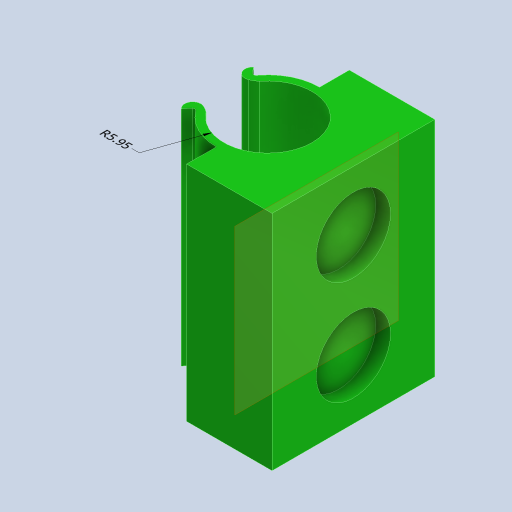
# Autodesk Inventor part: крепление маркера 11мм
Saved by Autodesk Inventor 2024.2 (Build 282272000, 272)
## iProperties
Created: 2025-12-12
Part Number: крепление маркера 11мм
Material: Типовые
Document SubType Name: Modeling
Designer: katya_notebook
Density: 1 g/cm^3
Appearance: Темно-зеленый
Author: katya_notebook
Autodesk Inventor part; units mm, degrees
ref_plane "YZ Plane" through (0, 0, 0) normal (1, 0, 0) x (0, 1, 0)
ref_plane "XZ Plane" through (0, 0, 0) normal (0, 1, 0) x (-1, 0, 0)
ref_plane "XY Plane" through (0, 0, 0) normal (0, 0, 1) x (1, 0, 0)
sketch "Эскиз1" plane through (0, 0, 0) normal (0, 1, 0) x (-1, 0, 0)
  circle A0 centre (0, 0) radius 5.95
  circle A1 centre (0, 0) radius 6.95
  line L0 (0, 0) -> (5.546, 4.1887)
  line L1 (0, 0) -> (5.546, -4.1887)
  point P0 (4.748, -3.586)
  point P1 (4.748, 3.586)
  dimension "d0" = 11.9
  dimension "d1" = 13.9
  constraints: 4 end point, 2 centre point, 2 coincident, 2 point on circle
  measures "d0" diameter of A0
  measures "d1" diameter of A1
extrude "Выдавливание1" add sketch "Эскиз1" along normal blind 30 contours A0 L1 A1 L0 picked at (4.878, 4.401)
sketch "Эскиз2" plane through (0, 30, 0) normal (0, 1, 0) x (1, 0, 0)
  arc A0 (-4.748, -3.586) -> (-5.6407, -3.0561) centre (-7.4493, -7.1199) ccw
  arc A1 (-5.6407, -3.0561) -> (-6.7976, -4.8618) centre (-6.075, -4.0513) ccw
  line L0 (-6.7976, -4.8618) -> (-6.1263, -4.0074)
  arc A2 (-5.5474, -4.1741) -> (-6.1263, -4.0074) centre (-5.9157, -4.3645) ccw
  line L1 (-4.748, -3.586) -> (-5.546, -4.1887)
  line L2 (-5.546, -4.1887) -> (-4.748, -3.586)
  line L3 (-5.546, -4.1887) -> (-5.5474, -4.1741)
  line L4 (-0.0151, 0) -> (-3.489, 0)
  arc A3 (-5.6407, 3.0561) -> (-4.748, 3.586) centre (-7.4493, 7.1199) ccw
  arc A4 (-6.1263, 4.0074) -> (-5.5474, 4.1741) centre (-5.9157, 4.3645) ccw
  line L5 (-4.748, 3.586) -> (-5.546, 4.1887)
  line L6 (-5.546, 4.1887) -> (-4.748, 3.586)
  line L7 (-5.546, 4.1887) -> (-5.5474, 4.1741)
  arc A5 (-6.7976, 4.8618) -> (-5.6407, 3.0561) centre (-6.075, 4.0513) ccw
  line L8 (-6.7976, 4.8618) -> (-6.1263, 4.0074)
  point P0 (-4.748, 3.586)
  point P1 (-5.546, -4.1887)
  point P2 (-5.3694, -4.0591)
  point P3 (-5.3694, 4.0591)
  dimension "d25" = 1.0859
  constraints: 18 end point, 12 point on circle, 12 symmetric about line, 6 centre point, 4 coincident, 1 collinear, 1 horizontal, 3 other
  measures "d25" radius of A1
sketch "Эскиз3" plane through (0, 30, 0) normal (0, 1, 0) x (1, 0, 0)
  arc A0 (-5.546, -4.1887) -> (-5.546, 4.1887) centre (0, 0) ccw projected
  line L0 (11.5, -6.95) -> (11.5, 6.95)
  arc A1 (-4.748, -3.586) -> (-4.748, 3.586) centre (0, 0) ccw projected
  line L1 (0, -6.95) -> (0, -5.95)
  line L2 (0, 5.95) -> (0, 6.95)
  line L3 (11.5, 6.95) -> (11.5, 10.95)
  line L4 (11.5, -6.95) -> (11.5, -10.95)
  line L5 (0, 2.45) -> (0, 6.95)
  line L6 (11.5, -10.95) -> (0, -10.95)
  line L7 (0, -10.95) -> (0, -6.95)
  line L8 (11.5, 10.95) -> (0, 10.95)
  line L9 (0, 10.95) -> (0, 6.95)
  arc A2 (0, -5.95) -> (0, 5.95) centre (0, 0) ccw
  dimension "d13" = 4
  dimension "d14" = 4
  dimension "d22" = 21.9
  dimension "d23" = 5
  constraints: 20 end point, 6 point on circle, 4 vertical, 2 horizontal, 2 perpendicular, 1 centre point, 1 collinear, 1 concentric
  measures "d13" distance of L4.end L0.start
  measures "d14" distance of L3.end L0.end
  measures "d22" distance of L4.end L3.end
  measures "d23" distance of L6.end L1.end
extrude "Выдавливание3" add sketch "Эскиз3" against normal blind 30
ref_plane "РабПлоскость1" through (11.5, 20, 4.95) normal (1, 0, 0) x (0, 0, -1)
sketch "Эскиз4" plane through (11.5, 20, 4.95) normal (1, 0, 0) x (0, 0, -1)
  line L0 (4.95, -20) -> (4.95, 10)
  line L1 (1, 10) -> (8.9, 10) projected
  circle A0 centre (4.95, -12) radius 5
  line L2 (14.4, -20) -> (-4.5, -20) projected
  circle A1 centre (4.95, 2) radius 5
  line L3 (-4.5, 10) -> (14.4, 10) projected
  point P0 (7.3306, 10)
  point P1 (2.5694, 10)
  point P2 (4.95, 10)
  dimension "d15" = 10
  dimension "d16" = 8
  dimension "d17" = 10
  dimension "d18" = 8
  constraints: 3 midpoint, 2 centre point, 2 end point, 2 point on line
  measures "d15" diameter of A0
  measures "d16" distance of A0.centre point (4.95, -20)
  measures "d17" diameter of A1
  measures "d18" distance of point (4.95, 10) A1.centre
extrude "Выдавливание4" cut sketch "Эскиз4" against normal blind 2
extrude "Выдавливание5" add sketch "Эскиз2" against normal blind 30
sketch "Эскиз5" plane through (0, 30, 0) normal (0, 1, 0) x (1, 0, 0)
  arc A0 (0, 6.95) -> (-5.546, 4.1887) centre (0, 0) ccw projected
  line L0 (-5.546, 4.1887) -> (-5.5474, 4.1741) projected
  arc A1 (-6.1263, 4.0074) -> (-5.5474, 4.1741) centre (-5.9157, 4.3645) ccw projected
  line L1 (-6.1263, 4.0074) -> (-6.7976, 4.8618) projected
  arc A2 (-6.7976, 4.8618) -> (-5.6407, 3.0561) centre (-6.075, 4.0513) ccw projected
  arc A3 (-5.6407, 3.0561) -> (-4.748, 3.586) centre (-7.4493, 7.1199) ccw projected
  arc A4 (-4.748, -3.586) -> (-4.748, 3.586) centre (0, 0) ccw projected
  arc A5 (-4.748, -3.586) -> (-5.6407, -3.0561) centre (-7.4493, -7.1199) ccw projected
  arc A6 (-5.6407, -3.0561) -> (-6.7976, -4.8618) centre (-6.075, -4.0513) ccw projected
  line L2 (-6.7976, -4.8618) -> (-6.1263, -4.0074) projected
  arc A7 (-5.5474, -4.1741) -> (-6.1263, -4.0074) centre (-5.9157, -4.3645) ccw projected
  line L3 (-5.5474, -4.1741) -> (-5.546, -4.1887) projected
  arc A8 (-5.546, -4.1887) -> (0, -6.95) centre (0, 0) ccw projected
  line L4 (0, -6.95) -> (0, -10.95) projected
  line L5 (0, -10.95) -> (11.5, -10.95) projected
  line L6 (11.5, -10.95) -> (11.5, 10.95) projected
  line L7 (11.5, 10.95) -> (0, 10.95) projected
  line L8 (0, 10.95) -> (0, 6.95) projected
  line L9 (0, 5.95) -> (0, 6.95)
  line L10 (0, -5.95) -> (0, -6.95)
  constraints: 4 end point, 2 point on circle, 1 collinear, 1 point on line, 1 vertical
extrude "Выдавливание6" [suppressed]
sketch "Эскиз6" plane through (11.5, 30, 10.95) normal (1, 0, 0) x (0, 0, -1)
  arc A0 (15.95, -22) -> (15.95, -22) centre (10.95, -22) ccw projected
  arc A1 (15.95, -8) -> (15.95, -8) centre (10.95, -8) ccw projected
  point P0 (10.95, -30)
extrude "Выдавливание7" [suppressed]
